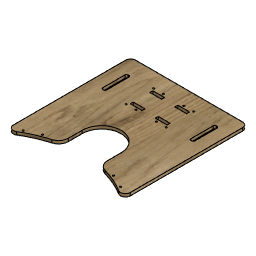
Partie_Haute_Plastique (Autodesk Fusion 360 archive; units mm, degrees)
design "Base_Robot"
Autodesk Fusion 360 part; units mm, degrees
sketch "Sketch1" plane through (0, 0, 0) normal (0, 0, 1) x (1, 0, 0)
  line L0 (-120, 175) -> (120, 175)
  line L1 (120, 175) -> (120, -175)
  line L2 (120, -175) -> (-120, -175)
  line L3 (-120, -175) -> (-120, 175)
  line L4 (-120, 175) -> (120, -175) construction
  line L5 (120, 175) -> (-120, -175) construction
  dimension "d1" = 240
  dimension "d2" = 350
  constraint horizontal L0
  constraint perpendicular L0 L1
  constraint parallel L0 L2
  constraint parallel L1 L3
  constraint coincident L4 origin
  constraint coincident L5 origin
  measures "d1" distance of L1.end L2.end
  measures "d2" distance of L0.end L1.end
extrude "Extrude1" add sketch "Sketch1" along normal blind 6
sketch "Sketch2" plane through (0, 0, 6) normal (0, 0, 1) x (-1, 0, 0)
  line L0 (120, 175) -> (-120, 175)
  line L1 (-120, 175) -> (-120, -175)
  line L2 (-120, -175) -> (120, -175)
  line L3 (120, -175) -> (120, 175)
  line L4 (0, -2.5) -> (0, -20)
  line L5 (37.6695, -98.197) -> (13.6695, -98.197)
  line L6 (13.6695, -98.197) -> (13.6695, -92.197)
  line L7 (13.6695, -92.197) -> (37.6695, -92.197)
  line L8 (37.6695, -92.197) -> (37.6695, -98.197)
  line L9 (-13.6695, -98.197) -> (-37.6695, -98.197)
  line L10 (-37.6695, -98.197) -> (-37.6695, -92.197)
  line L11 (-37.6695, -92.197) -> (-13.6695, -92.197)
  line L12 (-13.6695, -92.197) -> (-13.6695, -98.197)
  line L13 (13.6695, -98.197) -> (-13.6695, -98.197) construction
  line L14 (13.6695, -92.197) -> (0, 0) construction
  line L15 (0, 0) -> (-13.6695, -92.197) construction
  line L16 (37.6695, -138.291) -> (13.6695, -138.291)
  line L17 (13.6695, -138.291) -> (13.6695, -132.291)
  line L18 (13.6695, -132.291) -> (37.6695, -132.291)
  line L19 (37.6695, -132.291) -> (37.6695, -138.291)
  line L20 (-13.6695, -138.291) -> (-37.6695, -138.291)
  line L21 (-37.6695, -138.291) -> (-37.6695, -132.291)
  line L22 (-37.6695, -132.291) -> (-13.6695, -132.291)
  line L23 (-13.6695, -132.291) -> (-13.6695, -138.291)
  line L24 (13.6695, -132.291) -> (13.6695, -98.197) construction
  line L25 (-13.6695, -132.291) -> (-13.6695, -98.197) construction
  line L26 (13.6695, -132.291) -> (-13.6695, -132.291) construction
  circle A0 centre (40.9997, -143.3) radius 1.7
  circle A1 centre (21.0197, -143.3) radius 1.7
  line L27 (40.9997, -143.3) -> (21.0197, -143.3) construction
  circle A2 centre (40.9997, -87.188) radius 1.7
  circle A3 centre (21.0197, -87.188) radius 1.7
  line L28 (40.9997, -87.188) -> (21.0197, -87.188) construction
  line L29 (37.6695, -92.197) -> (40.0585, -88.6037) construction
  line L30 (40.9997, -87.188) -> (40.0585, -88.6037) construction
  line L31 (21.0197, -87.188) -> (21.0197, -88.888) construction
  line L32 (21.0197, -92.197) -> (21.0197, -88.888) construction
  line L33 (40.9997, -143.3) -> (40.0585, -141.8843) construction
  line L34 (40.0585, -141.8843) -> (37.6695, -138.291) construction
  line L35 (21.0197, -143.3) -> (21.0197, -141.6) construction
  line L36 (21.0197, -141.6) -> (21.0197, -138.291) construction
  circle A4 centre (-21.0197, -143.3) radius 1.7
  circle A5 centre (-40.9997, -143.3) radius 1.7
  line L37 (-21.0197, -143.3) -> (-40.9997, -143.3) construction
  line L38 (-21.0197, -143.3) -> (-21.0197, -141.6) construction
  line L39 (-21.0197, -138.291) -> (-21.0197, -141.6) construction
  line L40 (-40.9997, -143.3) -> (-40.0585, -141.8843) construction
  line L41 (-37.6695, -138.291) -> (-40.0585, -141.8843) construction
  circle A6 centre (-21.0197, -87.188) radius 1.7
  circle A7 centre (-40.9997, -87.188) radius 1.7
  line L42 (-21.0197, -87.188) -> (-40.9997, -87.188) construction
  line L43 (-40.9997, -87.188) -> (-40.0585, -88.6037) construction
  line L44 (-37.6695, -92.197) -> (-40.0585, -88.6037) construction
  line L45 (-21.0197, -87.188) -> (-21.0197, -88.888) construction
  line L46 (-21.0197, -92.197) -> (-21.0197, -88.888) construction
  dimension "d5" = 24
  dimension "d6" = 6
  dimension "d7" = 27.339
  dimension "d8" = 34.094
  dimension "d11" = 3.4
  dimension "d12" = 19.98
  dimension "d13" = 4.315
  dimension "d14" = 3.309
  dimension "d15" = 30
  constraint horizontal L5
  constraint vertical L6
  constraint horizontal L7
  constraint vertical L8
  constraint horizontal L9
  constraint vertical L10
  constraint horizontal L11
  constraint vertical L12
  constraint equal L6 L12
  constraint equal L5 L9
  constraint horizontal L13
  constraint coincident L14.end L15.start
  constraint equal L14 L15
  constraint horizontal L16
  constraint vertical L17
  constraint horizontal L18
  constraint vertical L19
  constraint horizontal L20
  constraint vertical L21
  constraint horizontal L22
  constraint vertical L23
  constraint equal L9 L22
  constraint equal L5 L18
  constraint equal L6 L17
  constraint equal L17 L23
  constraint vertical L25
  constraint vertical L24
  constraint horizontal L26
  constraint equal A0 A1
  constraint coincident A0.centre L27.start
  constraint coincident A1.centre L27.end
  constraint horizontal L27
  constraint coincident A2.centre L28.start
  constraint coincident A3.centre L28.end
  constraint horizontal L28
  constraint equal A2 A3
  constraint equal A0 A2
  constraint coincident A2 L29.end
  constraint parallel L29 L30
  constraint coincident A3 L31.end
  constraint perpendicular L28 L31
  constraint coincident L7 L32.start
  constraint perpendicular L7 L32
  constraint coincident A0 L33.end
  constraint parallel L33 L34
  constraint coincident A1 L35.end
  constraint perpendicular L27 L35
  constraint coincident L16 L36.end
  constraint perpendicular L16 L36
  constraint equal L32 L36
  constraint equal L29 L34
  constraint equal L27 L28
  constraint coincident A4.centre L37.start
  constraint coincident A5.centre L37.end
  constraint horizontal L37
  constraint coincident A4 L38.end
  constraint coincident L20 L39.start
  constraint perpendicular L20 L39
  constraint coincident A5 L40.end
  constraint parallel L40 L41
  constraint parallel L38 L39
  constraint equal A4 A5
  constraint equal A1 A4
  constraint equal L36 L39
  constraint equal L34 L41
  constraint equal L27 L37
  constraint coincident A6.centre L42.start
  constraint coincident A7.centre L42.end
  constraint parallel L11 L42
  constraint coincident A7 L43.end
  constraint coincident A6 L45.end
  constraint coincident L11 L46.start
  constraint parallel L43 L44
  constraint perpendicular L11 L46
  constraint parallel L45 L46
  constraint equal A3 A6
  constraint equal A6 A7
  constraint equal L32 L46
  constraint equal L29 L44
  constraint equal L28 L42
  measures "d5" distance of L5.start L5.end
  measures "d6" distance of L5.start L7.end
  measures "d7" distance of L5.end L9.start
  measures "d8" distance of L9 L22
  measures "d11" diameter of A0
  measures "d12" distance of A0.centre A1.centre
  measures "d13" distance of L16.start L33.end
  measures "d14" distance of L35.end L36.end
  measures "d15" distance of L2 A1
extrude "Extrude2" cut sketch "Sketch2" against normal up to surface (6 mm away) contours L5 L6 L7 L8 | L9 L10 L11 L12 | L16 L17 L18 L19 | L20 L21 L22 L23 | A0 | A1 | A2 | A3 | A4 | A5 | A6 | A7
sketch "Sketch4" plane through (0, 0, 6) normal (0, 0, 1) x (-1, 0, 0)
  circle A0 centre (-40.9997, -87.188) radius 1.7
  line L0 (37.6695, -132.291) -> (37.6695, -138.291)
  line L1 (37.6695, -138.291) -> (13.6695, -138.291)
  line L2 (13.6695, -138.291) -> (13.6695, -132.291)
  line L3 (13.6695, -132.291) -> (37.6695, -132.291)
  circle A1 centre (21.0197, -87.188) radius 1.7
  circle A2 centre (40.9997, -87.188) radius 1.7
  circle A3 centre (21.0197, -143.3) radius 1.7
  circle A4 centre (-40.9997, -143.3) radius 1.7
  circle A5 centre (-21.0197, -87.188) radius 1.7
  line L4 (-13.6695, -132.291) -> (-13.6695, -138.291)
  line L5 (-13.6695, -138.291) -> (-37.6695, -138.291)
  line L6 (-37.6695, -138.291) -> (-37.6695, -132.291)
  line L7 (-37.6695, -132.291) -> (-13.6695, -132.291)
  line L8 (37.6695, -92.197) -> (37.6695, -98.197)
  line L9 (37.6695, -98.197) -> (13.6695, -98.197)
  line L10 (13.6695, -98.197) -> (13.6695, -92.197)
  line L11 (13.6695, -92.197) -> (37.6695, -92.197)
  line L12 (-13.6695, -92.197) -> (-13.6695, -98.197)
  line L13 (-13.6695, -98.197) -> (-37.6695, -98.197)
  line L14 (-37.6695, -98.197) -> (-37.6695, -92.197)
  line L15 (-37.6695, -92.197) -> (-13.6695, -92.197)
  circle A6 centre (40.9997, -143.3) radius 1.7
  circle A7 centre (-21.0197, -143.3) radius 1.7
  line L16 (120, 175) -> (-120, 175)
  line L17 (-120, 175) -> (-120, -175)
  line L18 (-120, -175) -> (120, -175)
  line L19 (120, -175) -> (120, 175)
  line L20 (94.5005, -138.244) -> (94.5005, -92.244)
  line L21 (91.5005, -89.244) -> (89.5005, -89.244)
  line L22 (86.5005, -138.244) -> (86.5005, -92.244)
  line L23 (91.5005, -141.244) -> (89.5005, -141.244)
  arc A8 (91.5005, -141.244) -> (94.5005, -138.244) centre (91.5005, -138.244) ccw
  arc A9 (94.5005, -138.244) -> (91.5005, -141.244) centre (91.5005, -138.244) ccw construction
  arc A10 (86.5005, -138.244) -> (89.5005, -141.244) centre (89.5005, -138.244) ccw
  arc A11 (89.5005, -141.244) -> (86.5005, -138.244) centre (89.5005, -138.244) ccw construction
  arc A12 (89.5005, -89.244) -> (86.5005, -92.244) centre (89.5005, -92.244) ccw
  arc A13 (86.5005, -92.244) -> (89.5005, -89.244) centre (89.5005, -92.244) ccw construction
  arc A14 (94.5005, -92.244) -> (91.5005, -89.244) centre (91.5005, -92.244) ccw
  arc A15 (91.5005, -89.244) -> (94.5005, -92.244) centre (91.5005, -92.244) ccw construction
  line L24 (89.5005, -92.244) -> (40.9997, -87.188) construction
  line L25 (89.5005, -138.244) -> (40.9997, -143.3) construction
  dimension "d22" = 3
  dimension "d23" = 2
  dimension "d24" = 46
  dimension "d25" = 48.831
  constraint tangent L20 A14
  constraint tangent L21 A12
  constraint tangent L22 A12
  constraint tangent L23 A10
  constraint tangent L23 A8
  constraint tangent L20 A8
  constraint tangent L21 A14
  constraint tangent L22 A10
  constraint horizontal L23
  constraint horizontal L21
  constraint vertical L22
  constraint vertical L20
  constraint equal A10 A14
  constraint equal A12 A14
  constraint equal A8 A10
  constraint concentric A8 A9
  constraint concentric A10 A11
  constraint concentric A12 A13
  constraint concentric A14 A15
  constraint coincident A12.centre A13.centre
  constraint coincident A2.centre L24.end
  constraint coincident A10.centre A11.centre
  constraint coincident A6.centre L25.end
  constraint equal L24 L25
  measures "d22" radius of A8
  measures "d23" distance of L23.start L23.end
  measures "d24" distance of L22.start L22.end
  measures "d25" distance of L0 L22
extrude "Extrude3" cut sketch "Sketch4" against normal up to surface (6 mm away) contours L20 L21 L22 L23 A8 A10 A12 A14
mirror "Mirror1" about plane through (0, 0, 0) normal (1, 0, 0) of "Extrude3"
sketch "Sketch5" plane through (0, 0, 6) normal (0, 0, 1) x (-1, 0, 0)
  line L0 (-91.5005, -89.244) -> (-89.5005, -89.244)
  arc A0 (-86.5005, -92.244) -> (-89.5005, -89.244) centre (-89.5005, -92.244) ccw
  line L1 (-86.5005, -92.244) -> (-86.5005, -138.244)
  arc A1 (-89.5005, -141.244) -> (-86.5005, -138.244) centre (-89.5005, -138.244) ccw
  line L2 (-89.5005, -141.244) -> (-91.5005, -141.244)
  arc A2 (-94.5005, -138.244) -> (-91.5005, -141.244) centre (-91.5005, -138.244) ccw
  line L3 (-94.5005, -138.244) -> (-94.5005, -92.244)
  arc A3 (-91.5005, -89.244) -> (-94.5005, -92.244) centre (-91.5005, -92.244) ccw
  line L4 (86.5005, -138.244) -> (86.5005, -92.244)
  arc A4 (89.5005, -89.244) -> (86.5005, -92.244) centre (89.5005, -92.244) ccw
  line L5 (89.5005, -89.244) -> (91.5005, -89.244)
  arc A5 (94.5005, -92.244) -> (91.5005, -89.244) centre (91.5005, -92.244) ccw
  line L6 (94.5005, -92.244) -> (94.5005, -138.244)
  arc A6 (91.5005, -141.244) -> (94.5005, -138.244) centre (91.5005, -138.244) ccw
  line L7 (91.5005, -141.244) -> (89.5005, -141.244)
  arc A7 (86.5005, -138.244) -> (89.5005, -141.244) centre (89.5005, -138.244) ccw
  circle A8 centre (-40.9997, -87.188) radius 1.7
  line L8 (37.6695, -132.291) -> (37.6695, -138.291)
  line L9 (37.6695, -138.291) -> (13.6695, -138.291)
  line L10 (13.6695, -138.291) -> (13.6695, -132.291)
  line L11 (13.6695, -132.291) -> (37.6695, -132.291)
  circle A9 centre (21.0197, -87.188) radius 1.7
  circle A10 centre (40.9997, -87.188) radius 1.7
  circle A11 centre (21.0197, -143.3) radius 1.7
  circle A12 centre (-40.9997, -143.3) radius 1.7
  circle A13 centre (-21.0197, -87.188) radius 1.7
  line L12 (-13.6695, -132.291) -> (-13.6695, -138.291)
  line L13 (-13.6695, -138.291) -> (-37.6695, -138.291)
  line L14 (-37.6695, -138.291) -> (-37.6695, -132.291)
  line L15 (-37.6695, -132.291) -> (-13.6695, -132.291)
  line L16 (37.6695, -92.197) -> (37.6695, -98.197)
  line L17 (37.6695, -98.197) -> (13.6695, -98.197)
  line L18 (13.6695, -98.197) -> (13.6695, -92.197)
  line L19 (13.6695, -92.197) -> (37.6695, -92.197)
  line L20 (-13.6695, -92.197) -> (-13.6695, -98.197)
  line L21 (-13.6695, -98.197) -> (-37.6695, -98.197)
  line L22 (-37.6695, -98.197) -> (-37.6695, -92.197)
  line L23 (-37.6695, -92.197) -> (-13.6695, -92.197)
  circle A14 centre (40.9997, -143.3) radius 1.7
  circle A15 centre (-21.0197, -143.3) radius 1.7
  line L24 (120, 175) -> (-120, 175)
  line L25 (-120, 175) -> (-120, -175)
  line L26 (-120, -175) -> (120, -175)
  line L27 (120, -175) -> (120, 175)
  line L28 (0, -2.5) -> (0, -20)
  circle A16 centre (0, 4.512) radius 40
  line L29 (21.0197, -85.488) -> (-21.0197, -85.488) construction
  dimension "d30" = 80
  dimension "d31" = 50
  constraint coincident L28 A16.centre
  constraint coincident A9 L29.start
  constraint coincident A13 L29.end
  constraint tangent A13 L29
  constraint parallel L19 L29
  measures "d30" diameter of A16
  measures "d31" distance of A16 L29
extrude "Extrude4" cut sketch "Sketch5" against normal up to surface (6 mm away) contours A16
sketch "Sketch6" plane through (0, 0, 6) normal (0, 0, 1) x (-1, 0, 0)
  circle A0 centre (0, 4.512) radius 40 construction
  line L0 (-91.5005, -89.244) -> (-89.5005, -89.244)
  arc A1 (-86.5005, -92.244) -> (-89.5005, -89.244) centre (-89.5005, -92.244) ccw
  line L1 (-86.5005, -92.244) -> (-86.5005, -138.244)
  arc A2 (-89.5005, -141.244) -> (-86.5005, -138.244) centre (-89.5005, -138.244) ccw
  line L2 (-89.5005, -141.244) -> (-91.5005, -141.244)
  arc A3 (-94.5005, -138.244) -> (-91.5005, -141.244) centre (-91.5005, -138.244) ccw
  line L3 (-94.5005, -138.244) -> (-94.5005, -92.244)
  arc A4 (-91.5005, -89.244) -> (-94.5005, -92.244) centre (-91.5005, -92.244) ccw
  line L4 (86.5005, -138.244) -> (86.5005, -92.244)
  arc A5 (89.5005, -89.244) -> (86.5005, -92.244) centre (89.5005, -92.244) ccw
  line L5 (89.5005, -89.244) -> (91.5005, -89.244)
  arc A6 (94.5005, -92.244) -> (91.5005, -89.244) centre (91.5005, -92.244) ccw
  line L6 (94.5005, -92.244) -> (94.5005, -138.244)
  arc A7 (91.5005, -141.244) -> (94.5005, -138.244) centre (91.5005, -138.244) ccw
  line L7 (91.5005, -141.244) -> (89.5005, -141.244)
  arc A8 (86.5005, -138.244) -> (89.5005, -141.244) centre (89.5005, -138.244) ccw
  circle A9 centre (-40.9997, -87.188) radius 1.7
  line L8 (37.6695, -132.291) -> (37.6695, -138.291)
  line L9 (37.6695, -138.291) -> (13.6695, -138.291)
  line L10 (13.6695, -138.291) -> (13.6695, -132.291)
  line L11 (13.6695, -132.291) -> (37.6695, -132.291)
  circle A10 centre (21.0197, -87.188) radius 1.7
  circle A11 centre (40.9997, -87.188) radius 1.7
  circle A12 centre (21.0197, -143.3) radius 1.7
  circle A13 centre (-40.9997, -143.3) radius 1.7
  circle A14 centre (-21.0197, -87.188) radius 1.7
  line L12 (-13.6695, -132.291) -> (-13.6695, -138.291)
  line L13 (-13.6695, -138.291) -> (-37.6695, -138.291)
  line L14 (-37.6695, -138.291) -> (-37.6695, -132.291)
  line L15 (-37.6695, -132.291) -> (-13.6695, -132.291)
  line L16 (37.6695, -92.197) -> (37.6695, -98.197)
  line L17 (37.6695, -98.197) -> (13.6695, -98.197)
  line L18 (13.6695, -98.197) -> (13.6695, -92.197)
  line L19 (13.6695, -92.197) -> (37.6695, -92.197)
  line L20 (-13.6695, -92.197) -> (-13.6695, -98.197)
  line L21 (-13.6695, -98.197) -> (-37.6695, -98.197)
  line L22 (-37.6695, -98.197) -> (-37.6695, -92.197)
  line L23 (-37.6695, -92.197) -> (-13.6695, -92.197)
  circle A15 centre (40.9997, -143.3) radius 1.7
  circle A16 centre (-21.0197, -143.3) radius 1.7
  line L24 (120, 175) -> (-120, 175)
  line L25 (-120, 175) -> (-120, -175)
  line L26 (-120, -175) -> (120, -175)
  line L27 (120, -175) -> (120, 175)
  circle A17 centre (0, 244.512) radius 200
  circle A18 centre (0, 4.512) radius 40 construction
  line L28 (0, 244.512) -> (0, 4.512) construction
  line L29 (40, 48.5528) -> (40, 4.512)
  line L30 (40, 4.512) -> (-40, 4.512)
  line L31 (-40, 4.512) -> (-40, 48.5528)
  dimension "d34" = 400
  dimension "d40" = 80
  constraint coincident A17.centre L28.start
  constraint coincident A0.centre A18.centre
  constraint vertical L28
  constraint coincident A17 L29.start
  constraint coincident A0 L29.end
  constraint coincident A18 L30.end
  constraint coincident A17 L31.end
  constraint coincident A0.centre L30
  constraint vertical L29
  constraint vertical L31
  constraint horizontal L30
  measures "d34" diameter of A17
  measures "d40" distance of A0 A17
extrude "Extrude5" cut sketch "Sketch6" against normal up to surface (6 mm away) contours L24 L25 L27 A17 | A17 L29 L30 L31 picked at (-4.4713, 131.6541)
fillet "Fillet1" radius 20 2 edges at (-40, -48.5528, 3) (40, -48.5528, 3)
sketch "Sketch8" plane through (0, 0, 6) normal (0, 0, 1) x (-1, 0, 0)
  arc A0 (-40, 32.8519) -> (-54.5455, 52.0937) centre (-60, 32.8519) ccw
  arc A1 (-120, 84.512) -> (-54.5455, 52.0937) centre (0, 244.512) ccw
  line L0 (-120, 84.512) -> (-120, -175)
  line L1 (-120, -175) -> (120, -175)
  line L2 (120, -175) -> (120, 84.512)
  arc A2 (54.5455, 52.0937) -> (120, 84.512) centre (0, 244.512) ccw
  arc A3 (54.5455, 52.0937) -> (40, 32.8519) centre (60, 32.8519) ccw
  line L3 (40, 32.8519) -> (40, 4.512)
  arc A4 (-40, 4.512) -> (40, 4.512) centre (0, 4.512) ccw
  line L4 (-40, 4.512) -> (-40, 32.8519)
  line L5 (-91.5005, -89.244) -> (-89.5005, -89.244)
  arc A5 (-86.5005, -92.244) -> (-89.5005, -89.244) centre (-89.5005, -92.244) ccw
  line L6 (-86.5005, -92.244) -> (-86.5005, -138.244)
  arc A6 (-89.5005, -141.244) -> (-86.5005, -138.244) centre (-89.5005, -138.244) ccw
  line L7 (-89.5005, -141.244) -> (-91.5005, -141.244)
  arc A7 (-94.5005, -138.244) -> (-91.5005, -141.244) centre (-91.5005, -138.244) ccw
  line L8 (-94.5005, -138.244) -> (-94.5005, -92.244)
  arc A8 (-91.5005, -89.244) -> (-94.5005, -92.244) centre (-91.5005, -92.244) ccw
  line L9 (86.5005, -138.244) -> (86.5005, -92.244)
  arc A9 (89.5005, -89.244) -> (86.5005, -92.244) centre (89.5005, -92.244) ccw
  line L10 (89.5005, -89.244) -> (91.5005, -89.244)
  arc A10 (94.5005, -92.244) -> (91.5005, -89.244) centre (91.5005, -92.244) ccw
  line L11 (94.5005, -92.244) -> (94.5005, -138.244)
  arc A11 (91.5005, -141.244) -> (94.5005, -138.244) centre (91.5005, -138.244) ccw
  line L12 (91.5005, -141.244) -> (89.5005, -141.244)
  arc A12 (86.5005, -138.244) -> (89.5005, -141.244) centre (89.5005, -138.244) ccw
  circle A13 centre (-40.9997, -87.188) radius 1.7
  line L13 (37.6695, -132.291) -> (37.6695, -138.291)
  line L14 (37.6695, -138.291) -> (13.6695, -138.291)
  line L15 (13.6695, -138.291) -> (13.6695, -132.291)
  line L16 (13.6695, -132.291) -> (37.6695, -132.291)
  circle A14 centre (21.0197, -87.188) radius 1.7
  circle A15 centre (40.9997, -87.188) radius 1.7
  circle A16 centre (21.0197, -143.3) radius 1.7
  circle A17 centre (-40.9997, -143.3) radius 1.7
  circle A18 centre (-21.0197, -87.188) radius 1.7
  line L17 (-13.6695, -132.291) -> (-13.6695, -138.291)
  line L18 (-13.6695, -138.291) -> (-37.6695, -138.291)
  line L19 (-37.6695, -138.291) -> (-37.6695, -132.291)
  line L20 (-37.6695, -132.291) -> (-13.6695, -132.291)
  line L21 (37.6695, -92.197) -> (37.6695, -98.197)
  line L22 (37.6695, -98.197) -> (13.6695, -98.197)
  line L23 (13.6695, -98.197) -> (13.6695, -92.197)
  line L24 (13.6695, -92.197) -> (37.6695, -92.197)
  line L25 (-13.6695, -92.197) -> (-13.6695, -98.197)
  line L26 (-13.6695, -98.197) -> (-37.6695, -98.197)
  line L27 (-37.6695, -98.197) -> (-37.6695, -92.197)
  line L28 (-37.6695, -92.197) -> (-13.6695, -92.197)
  circle A19 centre (40.9997, -143.3) radius 1.7
  circle A20 centre (-21.0197, -143.3) radius 1.7
  arc A21 (55.9091, 47.2833) -> (123, 80.512) centre (0, 244.512) ccw construction
  circle A22 centre (100, 65.5567) radius 1.7
  circle A23 centre (72.8108, 52.878) radius 1.7
  dimension "d45" = 5
  dimension "d46" = 3.4
  dimension "d47" = 30
  dimension "d48" = 20
  constraint coincident A21 A22.centre
  constraint coincident A21 A23.centre
  constraint equal A22 A23
  measures "d46" diameter of A23
  measures "d47" distance of A22.centre A23.centre
  measures "d48" distance of L2 A22.centre
extrude "Extrude7" cut sketch "Sketch8" against normal up to surface (6 mm away) contours A22 | A23
mirror "Mirror2" about plane through (0, 0, 0) normal (1, 0, 0) of "Extrude7"
fillet "Fillet2" radius 10 4 edges at (120, -84.512, 3) (120, 175, 3) (-120, 175, 3) (-120, -84.512, 3)
